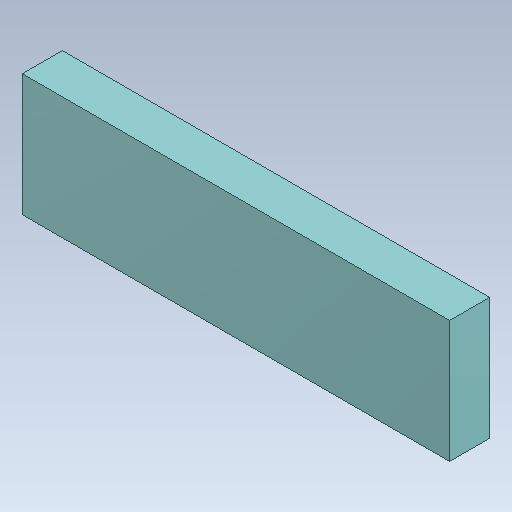
# Autodesk Inventor part: JTAG_SERIAL
Saved by Autodesk Inventor 2021 (Build 250183000, 183)
## iProperties
Created: 2020-11-03
Part Number: JTAG_SERIAL
Material: Generic
Document SubType Name: Modeling
Designer: faiya
Density: 1 g/cm^3
Appearance: JTAG_SERIAL_PTH, JTAG_SERIAL
Author: faiya
Autodesk Inventor part; units mm, degrees
ref_plane "YZ Plane" through (0, 0, 0) normal (1, 0, 0) x (0, 1, 0)
ref_plane "XZ Plane" through (0, 0, 0) normal (0, 1, 0) x (-1, 0, 0)
ref_plane "XY Plane" through (0, 0, 0) normal (0, 0, 1) x (1, 0, 0)
sketch "JTAG_SERIAL_PTH, JTAG_SERIAL_48" plane through (0, 0, 0) normal (0, 0, 1) x (1, 0, 0)
  line L0 (-5.334, 1.524) -> (5.334, 1.524)
  line L1 (5.334, 1.524) -> (5.334, -1.524)
  line L2 (5.334, -1.524) -> (-5.334, -1.524)
  line L3 (-5.334, -1.524) -> (-5.334, 1.524)
  constraints: 8 end point
extrude "Extrusion1" add sketch "JTAG_SERIAL_PTH, JTAG_SERIAL_48" along normal blind 1
body "Solid1"
